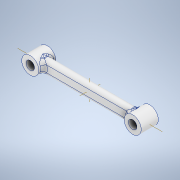
# Autodesk Inventor part: connecting rod
Saved by Autodesk Inventor 2021.1 (Build 251245000, 245)
## iProperties
Created: 2020-08-30
Part Number: connecting rod
Material: Aluminum 6061
Document SubType Name: Sheet Metal
Designer: Vamshi
Mass: 117.563 g
Surface Area: 139.323 cm^2
Volume: 43.5419 cm^3
Density: 2.7 g/cm^3
Sheet Metal Rule: Default
Appearance: Aluminum - Flat
Author: Vamshi
Autodesk Inventor part; units mm, degrees
ref_plane "YZ Plane" through (0, 0, 0) normal (1, 0, 0) x (0, 1, 0)
ref_plane "XZ Plane" through (0, 0, 0) normal (0, 1, 0) x (-1, 0, 0)
ref_plane "XY Plane" through (0, 0, 0) normal (0, 0, 1) x (1, 0, 0)
sketch "Sketch1" plane through (0, 0, 0) normal (0, 0, 1) x (1, 0, 0)
  circle A0 centre (-76.2, 0) radius 12.7
  circle A1 centre (-76.2, 0) radius 6.35
  circle A2 centre (76.2, 0) radius 12.7
  circle A3 centre (76.2, 0) radius 6.35
  line L0 (0, -17.78) -> (0, 17.78) projected
  point P0 (0, 0)
  dimension "d0" = 25.4
  dimension "d1" = 12.7
  dimension "d2" = 25.4
  dimension "d3" = 12.7
  dimension "d4" = 152.4
  constraints: 4 centre point, 2 coincident, 1 symmetric about line
  measures "d0" diameter of A0
  measures "d1" diameter of A1
  measures "d2" diameter of A2
  measures "d3" diameter of A3
  measures "d4" distance of A2.centre A0.centre
extrude "Extrusion1" add sketch "Sketch1" along normal mid plane 25.4
sketch "Sketch2" plane through (0, 0, 0) normal (0, 0, 1) x (1, 0, 0)
  circle A0 centre (-76.2, 0) radius 12.7 projected
  circle A1 centre (76.2, 0) radius 12.7 projected
  line L0 (-68.58, 10.16) -> (68.58, 10.16)
  line L1 (-68.58, -10.16) -> (68.58, -10.16)
  line L2 (-124.46, 0) -> (124.46, 0) projected
  point P0 (0, 0)
  point P1 (63.5, 0)
  point P2 (-63.5, 0)
  dimension "d7" = 20.32
  constraints: 4 end point, 4 point on circle, 2 horizontal, 1 other
  measures "d7" distance between parallel lines of L1 L0
extrude "Extrusion2" add sketch "Sketch2" along normal mid plane 10.16 contours L2 A1 L1 A0 | A0 L0 A1 L2
fillet "Fillet1" radius 10.16 6 edges at (-68.58, -10.16, 2.54) (-68.58, -10.16, -2.54) (68.58, -10.16, 0) (68.58, 10.16, 0) (-68.58, 10.16, 2.54) (-68.58, 10.16, -2.54)
fillet "Fillet2" radius 5.08 12 edges at (-68.122, 10.4463, 5.08) (68.122, 10.4463, 5.08) (0, 10.16, 5.08) (68.122, -10.4463, 5.08) (-68.122, -10.4463, 5.08) (0, -10.16, 5.08) (-68.122, -10.4463, -5.08) (68.122, -10.4463, -5.08) (0, -10.16, -5.08) (68.122, 10.4463, -5.08) (-68.122, 10.4463, -5.08) (0, 10.16, -5.08)
fillet "Fillet3" radius 5.08 22 edges at (-65.1174, -6.2021, -4.9545) (-68.0344, -9.7269, -2.5414) (-65.1174, 6.2021, -4.9545) (-68.0344, 9.7269, -2.5414) (-63.7679, -2.5947, -5.08) (-63.7679, 2.5947, -5.08) (-65.1174, 6.2021, 4.9545) (-68.0344, 9.7269, 2.5414) (-65.1174, -6.2021, 4.9545) (-68.0344, -9.7269, 2.5414) (-63.7679, -2.5947, 5.08) (-63.7679, 2.5947, 5.08) (65.1174, 6.2021, -4.9545) (68.0344, 9.7269, -2.5414) (65.1174, -6.2021, -4.9545) (68.0344, -9.7269, -2.5414) (63.5, 0, -5.08) (65.1174, -6.2021, 4.9545) (68.0344, -9.7269, 2.5414) (65.1174, 6.2021, 4.9545) (68.0344, 9.7269, 2.5414) (63.5, 0, 5.08)
equation "\"BendRadius\" = Thickness"
equation "\"BendReliefWidth\" = Thickness"
equation "\"BendReliefDepth\" = 0.5 * Thickness"
equation "\"CornerReliefSize\" = 4 * Thickness"
equation "\"MinimumRemnant\" = 2 * Thickness"
equation "\"TransitionRadius\" = BendRadius"
equation "\"JacobiRadiusSize\" = BendRadius"
equation "\"GapSize\" = Thickness"
equation "\"Thickness\" = 3.048"
body "Solid1"
